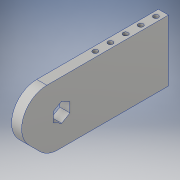
# Autodesk Inventor part: Pivot Plate
Saved by Autodesk Inventor 2019.4 (Build 234330000, 330)
## iProperties
Created: 2020-01-06
Part Number: Pivot Plate
Material: Aluminum 6061
Document SubType Name: Modeling
Designer: admin
Density: 2.7 g/cm^3
Appearance: Aluminum - Flat
Mass: 250.673 g
Surface Area: 294.361 cm^2
Volume: 92.8419 cm^3
Author: admin
Autodesk Inventor part; units mm, degrees
ref_plane "YZ Plane" through (0, 0, 0) normal (1, 0, 0) x (0, 1, 0)
ref_plane "XZ Plane" through (0, 0, 0) normal (0, 1, 0) x (-1, 0, 0)
ref_plane "XY Plane" through (0, 0, 0) normal (0, 0, 1) x (1, 0, 0)
sketch "Sketch1" plane through (0, 0, 0) normal (1, 0, 0) x (0, 1, 0)
  line L0 (-30.5, 90) -> (30.5, 90)
  line L1 (30.5, 90) -> (30.5, -90)
  line L2 (30.5, -90) -> (-30.5, -90)
  line L3 (-30.5, -90) -> (-30.5, 90)
  line L4 (-30.5, 90) -> (30.5, -90) construction
  line L5 (30.5, 90) -> (-30.5, -90) construction
  point P0 (0, 0)
  dimension "d0" = 61
  dimension "d1" = 180
  constraints: 12 end point, 2 midpoint, 2 parallel, 1 horizontal, 1 perpendicular
  measures "d0" distance of L1.end L2.end
  measures "d1" distance of L0.end L1.end
extrude "Extrusion1" add sketch "Sketch1" along normal mid plane 10
sketch "Sketch2" plane through (-5, 30.5, 90) normal (0, 1, 0) x (1, 0, 0)
  circle A0 centre (5, 172.5) radius 2.5
  circle A1 centre (5, 157.5) radius 2.5
  circle A2 centre (5, 142.5) radius 2.5
  circle A3 centre (5, 127.5) radius 2.5
  circle A4 centre (5, 112.5) radius 2.5
  line L0 (10, 180) -> (0, 180) projected
  line L1 (10, 180) -> (10, 0) projected
  point P0 (5, 90)
  dimension "d4" = 5
  dimension "d5" = 5
  dimension "d6" = 5
  dimension "d7" = 5
  dimension "d9" = 15
  dimension "d10" = 15
  dimension "d11" = 15
  dimension "d12" = 5
  dimension "d13" = 15
  dimension "d14" = 7.5
  dimension "d15" = 5
  dimension "d16" = 5
  dimension "d17" = 5
  dimension "d18" = 5
  dimension "d19" = 5
  constraints: 5 centre point
  measures "d4" diameter of A0
  measures "d5" diameter of A1
  measures "d6" diameter of A2
  measures "d7" diameter of A3
  measures "d9" distance of A2.centre A1.centre
  measures "d10" distance of A3.centre A2.centre
  measures "d11" distance of A0.centre A1.centre
  measures "d12" diameter of A4
  measures "d13" distance of A3.centre A4.centre
  measures "d14" distance from line of L0 A0.centre
  measures "d15" distance from line of L1 A4.centre
  measures "d16" distance from line of L1 A3.centre
  measures "d17" distance from line of L1 A2.centre
  measures "d18" distance from line of L1 A1.centre
  measures "d19" distance from line of L1 A0.centre
extrude "Extrusion2" cut sketch "Sketch2" against normal through all
sketch "Sketch3" plane through (5, 0, 0) normal (1, 0, 0) x (0, 0, -1)
  arc A0 (52.4343, -57.4151) -> (52.4343, -57.4151) centre (-15.9415, -0.6) ccw
  line L0 (-15.9415, 30.5) -> (-15.9415, -30.5) construction
  line L1 (90, -30.5) -> (-90, -30.5) projected
  arc A1 (-15.9415, 30.5) -> (-15.9415, -30.5) centre (-15.9415, 0) ccw construction
  line L2 (-90, 30.5) -> (-90, -30.5) projected
  line L3 (-90, -30.5) -> (90, -30.5) projected
  line L4 (90, -30.5) -> (90, 30.5) projected
  line L5 (90, 30.5) -> (-90, 30.5) projected
  arc A2 (-15.9415, -30.5) -> (-15.9415, 30.5) centre (-15.9415, 0) ccw construction
  line L6 (-15.9415, 9.5) -> (-7.7143, 4.75)
  line L7 (-7.7143, 4.75) -> (-7.7143, -4.75)
  line L8 (-7.7143, -4.75) -> (-15.9415, -9.5)
  line L9 (-15.9415, -9.5) -> (-24.1688, -4.75)
  line L10 (-24.1688, -4.75) -> (-24.1688, 4.75)
  line L11 (-24.1688, 4.75) -> (-15.9415, 9.5)
  point P0 (0, 0)
  dimension "d29" = 19
  constraints: 14 end point, 5 point on line, 4 point on circle, 2 centre point, 1 coincident, 1 midpoint, 1 vertical, 19 other
  measures "d29" distance of L7.end L10.end
extrude "Extrusion3" cut sketch "Sketch3" against normal through all contours L6 L7 L8 L9 L10 L11
chamfer "Chamfer1" distance 60 angle 45 1 edges at (0, -30.5, 90)
fillet "Fillet1" radius 25 3 edges at (0, 29.5, 90) (0, 30.5, 90) (0, -30.5, 30)
body "Solid1"
